leveler v1 (Autodesk Fusion 360 design; units mm, degrees)
Autodesk Fusion 360 part; units mm, degrees
sketch "Sketch1" plane through (0, 0, 0) normal (0, 0, 1) x (1, 0, 0)
  circle A0 centre (0, 0) radius 185
  circle A1 centre (0, 0) radius 186.2
  circle A2 centre (0, 0) radius 150
  circle A3 centre (0, 0) radius 100
  circle A4 centre (0, 0) radius 62.5
  circle A5 centre (0, 0) radius 15
  circle A6 centre (0, 0) radius 151.2
  circle A7 centre (0, 0) radius 101.2
  circle A8 centre (0, 0) radius 63.7
  circle A9 centre (0, 0) radius 16.2
  line L0 (0, 0) -> (0, 186.2) construction
  line L1 (-0.6, 184.999) -> (-0.6, 16.1889)
  line L2 (0.6, 16.1889) -> (0.6, 184.999)
  line L3 (-15.2111, 5.5733) -> (-175.7591, 57.7385)
  line L4 (-176.1299, 56.5972) -> (-15.582, 4.432)
  line L5 (-10.001, -12.7444) -> (-109.2251, -149.3147)
  line L6 (-108.2543, -150.02) -> (-9.0302, -13.4498)
  line L7 (9.0302, -13.4498) -> (108.2543, -150.02)
  line L8 (109.2251, -149.3147) -> (10.001, -12.7444)
  line L9 (15.582, 4.432) -> (176.1299, 56.5972)
  line L10 (175.7591, 57.7385) -> (15.2111, 5.5733)
  dimension "d1" = 370
  dimension "d2" = 1.2
  dimension "d3" = 300
  dimension "d4" = 200
  dimension "d5" = 125
  dimension "d6" = 30
  dimension "d7" = 1.2
  dimension "d8" = 1.2
  dimension "d9" = 1.2
  dimension "d10" = 1.2
  dimension "d11" = 1.2
  dimension "d13" = 360
  constraint coincident A0.centre A1.centre
  constraint concentric A0 A2
  constraint concentric A0 A3
  constraint concentric A3 A4
  constraint concentric A0 A5
  constraint coincident A1 L0.end
  constraint vertical L0
  constraint coincident A0 L1.start
  constraint coincident A9 L1.end
  constraint coincident A9 L2.start
  constraint coincident A0 L2.end
  constraint parallel L0 L2
  constraint parallel L0 L1
  measures "d1" diameter of A0
  measures "d3" diameter of A2
  measures "d4" diameter of A3
  measures "d5" diameter of A4
  measures "d6" diameter of A5
  measures "d11" distance of L1 L2
extrude "Extrude1" add sketch "Sketch1" along normal blind 0.3 contours A0 A6 L9 L10 | A0 A6 L7 L8 | A2 A6 L9 L10 | A2 A6 L8 L9 | A2 A6 L7 L8 | A0 A6 L1 L2 | A2 A6 L2 L10 | A2 A7 L9 L10 | A0 A6 L5 L6 | A2 A6 L6 L7 | A2 A7 L7 L8 | A2 A6 L1 L2 | A3 A7 L9 L10 | A3 A7 L8 L9 | A2 A6 L5 L6 | A3 A7 L7 L8 | A0 A6 L3 L4 | A2 A6 L1 L3 | A2 A7 L1 L2 | A3 A7 L2 L10 | A3 A8 L9 L10 | A2 A6 L4 L5 | A2 A7 L5 L6 | A3 A7 L6 L7 | A3 A8 L7 L8 | A2 A6 L3 L4 | A3 A7 L1 L2 | A4 A8 L9 L10 | A4 A8 L8 L9 | A3 A7 L5 L6 | A4 A8 L7 L8 | A2 A7 L3 L4 | A3 A7 L1 L3 | A3 A8 L1 L2 | A4 A8 L2 L10 | A4 A9 L9 L10 | A3 A7 L4 L5 | A3 A8 L5 L6 | A4 A8 L6 L7 | A4 A9 L7 L8 | A3 A7 L3 L4 | A4 A8 L1 L2 | A9 | A4 A8 L5 L6 | A3 A8 L3 L4 | A4 A8 L1 L3 | A4 A9 L1 L2 | A4 A8 L4 L5 | A4 A9 L5 L6 | A4 A8 L3 L4 | A4 A9 L3 L4 | A1
